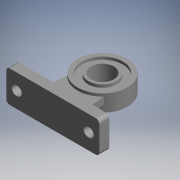
# Autodesk Inventor part: PDRHN50_b
Saved by Autodesk Inventor 2017.3 (Build 213256000, 256)
## iProperties
Part Number: PDRHN50_b
Material: Generic
Catalog Web Link: www.cadenas.de
Description: PDRH,PDRHN_body-Ball Bearing Units -High-Centered Pillow Type-
Vendor: MISUMI
Document SubType Name: Modeling
Designer: partserver
Manufacturer: MISUMI
Mass: 620.681 g
Surface Area: 931.576 cm^2
Volume: 620.681 cm^3
Density: 1 g/cm^3
Appearance: PSOLRGB-175-175-175
Category: PARTsolutions
Company: MISUMI
Title: PDRHN50
Author: Cadenas PARTsolutions
Comments: Ball Bearing Units -High-Centered Pillow Type-
PSOL_IDENT_0: {$CADENAS_DATA\23d-libs\misumi\metric\12_bearing_holders\pdrh\pdrh_body.prj},168 {VTYP=3D},{NB=PDRHN
PSOL_IDENT_1: 50_b},{LINA=PDRHN50},{NN=PDRH,PDRHN_body},{DATE=11.12.2019 10:04:59},{GEOMDATE=02.12.2019 07:12:02},
PSOL_IDENT_2: {VERSION=},{LINEID=100},{WBVAR=TS},{WBNUMERIC=}  {NB=PDRHN50_b},{LINA=PDRHN50},{KT=DUMMY},{PN=PDRHN5
PSOL_IDENT_3: 0},{TYPE=PDRHN},{MATH=Cast Iron Class No.30},{MATB=52100 Bearing Steel},{MATRS=Nitrile Rubber},{MATS
PSOL_IDENT_4: S=4137 Alloy Steel},{PRECISION=JIS B 1558/JIS B 1514/JIS B 1559},{OT=-15 ~+100},{TS=2},{TSALG='1','L
PSOL_IDENT_5: ubrication Type' , '2','Oil-Free Type'},{D=50},{JIS=UC210D1},{H=110},{L=206},{L1=159},{A=70},{DD1=22
PSOL_IDENT_6: },{DD=20},{TT=22},{H1=165},{B=51.6},{S=19.0},{CR=35.0},{COR=23.20},{M1=M8x1.0},{MD=8},{MPITCH=1.00},
PSOL_IDENT_7: {ML=10},{MASS=3900},{RLD1=110},{RLD2=90},{RLD3=62.4},{LD1=37},{LD2=6.0},{LD3=3},{G1=40.5},{G2=15.5},
PSOL_IDENT_8: {G3=55},{R1=16},{R2=8},{NCL=1.5},{KCL=23.6}
NB: PDRHN50_b
NN: PDRH,PDRHN_body
NT: Ball Bearing Units -High-Centered Pillow Type-
NBSYN: $PN._b
LINA: PDRHN50
CATALOG: Misumi
PN: PDRHN50
TYPE: PDRHN
MATH: Cast Iron Class No.30
MATB: 52100 Bearing Steel
MATRS: Nitrile Rubber
MATSS: 4137 Alloy Steel
PRECISION: JIS B 1558/JIS B 1514/JIS B 1559
OT: -15 ~+100
TS: Oil-Free Type
D: 50
JIS: UC210D1
H: 110
L: 206
L1: 159
A: 70
DD1: 22
DD: 20
TT: 22
H1: 165
B: 51.6
S: 19
CR: 35
COR: 23.2
M1: M8x1.0
MASS: 3900
SUPPLIER: MISUMI
ARTICLENO: PDRHN50_b
BOMINFO: PDRHN50
CREATOR: CADENAS GmbH
Autodesk Inventor part; units mm, degrees
sketch "_____3" plane through (0, 0, -18.5) normal (0, 0, 1) x (1, 0, 0)
  line L0 (-59.6047, 22) -> (59.6047, 22)
  arc A0 (43.6655, 36.6055) -> (59.6047, 22) centre (59.6047, 38) ccw
  line L1 (43.6655, 36.6055) -> (40.5, 72.7878)
  arc A1 (40.5, 72.7878) -> (-40.5, 72.7878) centre (0, 110) ccw
  line L2 (-40.5, 72.7878) -> (-43.6655, 36.6055)
  arc A2 (-59.6047, 22) -> (-43.6655, 36.6055) centre (-59.6047, 38) ccw
  constraints: 6 end point, 6 point on circle, 3 centre point
extrude "Extrusion1" add sketch "_____3" along normal blind 53.5
sketch "_____8" plane through (0, 0, 0) normal (1, 0, 0) x (0, 0, -1)
  line L0 (-35, 57.5488) -> (-35, 22)
  line L1 (-35, 22) -> (-18.5, 55)
  line L2 (-18.5, 55) -> (-18.5, 57.5488)
  line L3 (-18.5, 57.5488) -> (-35, 57.5488)
  constraints: 8 end point
extrude "Extrusion2" cut sketch "_____8" along normal mid plane 31
sketch "_____9" plane through (0, 0, 0) normal (1, 0, 0) x (0, 0, -1)
  line L0 (-18.5, 110) -> (-35, 110)
  line L1 (-35, 110) -> (-35, 165)
  line L2 (-35, 165) -> (-18.5, 165)
  line L3 (-18.5, 165) -> (-18.5, 110)
  line L4 (-18.5, 110) -> (-35, 110)
  constraints: 10 end point
revolve "Revolution1" cut sketch "_____9" angle 360 about axis through (0, 110, 18.5) along (0, 0, -1)
sketch "_____5" plane through (0, 0, 35) normal (0, 0, 1) x (1, 0, 0)
  line L0 (-65, 110) -> (-65, 0)
  line L1 (-65, 0) -> (65, 0)
  line L2 (65, 0) -> (65, 110)
  line L3 (65, 110) -> (55, 110)
  arc A0 (7.75, 55.5488) -> (55, 110) centre (0, 110) ccw
  line L4 (7.75, 55.5488) -> (7.75, 22)
  line L5 (7.75, 22) -> (-7.75, 22)
  line L6 (-7.75, 22) -> (-7.75, 55.5488)
  arc A1 (-55, 110) -> (-7.75, 55.5488) centre (0, 110) ccw
  line L7 (-55, 110) -> (-65, 110)
  constraints: 16 end point, 4 point on circle, 2 centre point
extrude "Extrusion3" cut sketch "_____5" against normal blind 32
sketch "_____6" plane through (0, 0, -18.5) normal (0, 0, 1) x (1, 0, 0)
  line L0 (-65, 110) -> (-65, 0)
  line L1 (-65, 0) -> (65, 0)
  line L2 (65, 0) -> (65, 110)
  line L3 (65, 110) -> (55, 110)
  arc A0 (-55, 110) -> (55, 110) centre (0, 110) ccw
  line L4 (-55, 110) -> (-65, 110)
  constraints: 10 end point, 2 point on circle, 1 centre point
extrude "Extrusion4" cut sketch "_____6" along normal blind 6
sketch "_____4" plane through (0, 0, 0) normal (0, 1, 0) x (1, 0, 0)
  line L0 (-103, 27) -> (-103, -27)
  arc A0 (-103, -27) -> (-95, -35) centre (-95, -27) ccw
  line L1 (-95, -35) -> (95, -35)
  arc A1 (95, -35) -> (103, -27) centre (95, -27) ccw
  line L2 (103, -27) -> (103, 27)
  arc A2 (103, 27) -> (95, 35) centre (95, 27) ccw
  line L3 (95, 35) -> (-95, 35)
  arc A3 (-95, 35) -> (-103, 27) centre (-95, 27) ccw
  constraints: 8 end point, 8 point on circle, 4 centre point
extrude "Extrusion5" add sketch "_____4" along normal blind 22
sketch "_____7" plane through (0, 0, 0) normal (0, 1, 0) x (1, 0, 0)
  arc A0 (78.5, 10) -> (78.5, -10) centre (78.5, 0) ccw
  line L0 (78.5, -10) -> (80.5, -10)
  arc A1 (80.5, -10) -> (80.5, 10) centre (80.5, 0) ccw
  line L1 (80.5, 10) -> (78.5, 10)
  constraints: 4 end point, 4 point on circle, 2 centre point
extrude "Extrusion6" cut sketch "_____7" along normal blind 22
sketch "_____10" plane through (0, 0, 0) normal (0, 1, 0) x (1, 0, 0)
  arc A0 (-80.5, 10) -> (-80.5, -10) centre (-80.5, 0) ccw
  line L0 (-80.5, -10) -> (-78.5, -10)
  arc A1 (-78.5, -10) -> (-78.5, 10) centre (-78.5, 0) ccw
  line L1 (-78.5, 10) -> (-80.5, 10)
  constraints: 4 end point, 4 point on circle, 2 centre point
extrude "Extrusion7" cut sketch "_____10" along normal blind 22
sketch "_____11" plane through (0, 0, 0) normal (1, 0, 0) x (0, 0, -1)
  line L0 (-12.5, 110) -> (-18.5, 110)
  line L1 (-18.5, 110) -> (-18.5, 155)
  line L2 (-18.5, 155) -> (-12.5, 155)
  line L3 (-12.5, 155) -> (-12.5, 110)
  line L4 (-12.5, 110) -> (-18.5, 110)
  constraints: 10 end point
revolve "Revolution2" cut sketch "_____11" angle 360 about axis through (0, 110, 12.5) along (0, 0, -1)
sketch "Sketch10" plane through (0, 110, -18.5) normal (0, 0, -1) x (-1, 0, 0)
  point P0 (0, 0)
hole "Hole1" at (0, 110, -18.5) direction (0, 0, 1) diameter 90 depth 6
sketch "_____13" plane through (0, 0, 0) normal (1, 0, 0) x (0, 0, -1)
  line L0 (19, 110) -> (-32.6, 110)
  line L1 (-32.6, 110) -> (-32.6, 141.2)
  line L2 (-32.6, 141.2) -> (19, 141.2)
  line L3 (19, 141.2) -> (19, 110)
  line L4 (19, 110) -> (-32.6, 110)
  constraints: 10 end point
revolve "Revolution3" add sketch "_____13" angle 360 about axis through (0, 110, -19) along (0, 0, -1)
sketch "Sketch12" plane through (0, 110, -19) normal (0, 0, -1) x (-1, 0, 0)
  point P0 (0, 0)
hole "Hole2" at (0, 110, -19) direction (0, 0, 1) diameter 50 depth 51.6
sketch "_____15" plane through (0, 0, 23.6) normal (0, 0, 1) x (1, 0, 0)
  line L0 (0, 110) -> (0, 141.2)
  line L1 (0, 141.2) -> (4, 141.2)
  line L2 (4, 141.2) -> (3.4585, 140.6585)
  line L3 (3.4585, 140.6585) -> (3.4585, 110)
  line L4 (3.4585, 110) -> (0, 110)
  line L5 (0, 110) -> (0, 141.2)
  constraints: 12 end point
revolve "Revolution4" cut sketch "_____15" angle 360 about axis through (0, 110, 23.6) along (0, -1, 0)
thread "Thread1" size "M8x1" class "6H" standard "ISO Metric profile" length 5.6585
sketch "_____16" plane through (0, 0, 23.6) normal (0, 0, 1) x (1, 0, 0)
  line L0 (0, 110) -> (-27.02, 94.4)
  line L1 (-27.02, 94.4) -> (-29.02, 97.8641)
  line L2 (-29.02, 97.8641) -> (-28.2803, 97.6659)
  line L3 (-28.2803, 97.6659) -> (-1.7292, 112.9951)
  line L4 (-1.7292, 112.9951) -> (0, 110)
  line L5 (0, 110) -> (-27.02, 94.4)
  constraints: 12 end point
revolve "Revolution5" cut sketch "_____16" angle 360 about axis through (0, 110, 23.6) along (0.8660254, 0.5, 0)
thread "Thread2" size "M8x1" class "6H" standard "ISO Metric profile" length 5.6585
ref_plane "CP1_XY" through (0, 135, 23.6) normal (0, 1, 0) x (1, 0, 0)
ref_plane "CP1_YZ" through (0, 135, 23.6) normal (1, 0, 0) x (0, 0, -1)
ref_plane "CP1_ZX" through (0, 135, 23.6) normal (0, 0, -1) x (0, 1, 0)
ref_plane "CP2_XY" through (-21.6506, 97.5, 23.6) normal (-0.8660254, -0.5, 0) x (-0.5, 0.8660254, 0)
ref_plane "CP2_YZ" through (-21.6506, 97.5, 23.6) normal (-0.5, 0.8660254, 0) x (0, 0, -1)
ref_plane "CP2_ZX" through (-21.6506, 97.5, 23.6) normal (0, 0, -1) x (-0.8660254, -0.5, 0)
body "Solid1"
